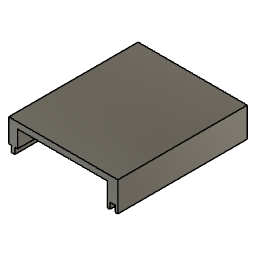
Headstage_dust_cover (Autodesk Fusion 360 design; units mm, degrees)
Autodesk Fusion 360 part; units mm, degrees
sketch "Sketch1" plane through (0, 22, 0) normal (0, 1, 0) x (-1, 0, 0)
  line L0 (11.5698, 0.25) -> (15.3, 0.25)
  line L1 (15.3, 0.25) -> (15.3, -0.5)
  line L2 (15.3, -0.5) -> (15.6004, -0.5)
  line L3 (15.6004, -0.5) -> (15.6004, -1.2)
  line L4 (15.6004, -1.2) -> (16.0004, -1.2)
  line L5 (16.0004, -1.2) -> (16.0004, -0.5)
  line L6 (16.0004, -0.5) -> (16.3, -0.5)
  line L7 (16.3, -0.5) -> (16.3, 1.05)
  line L8 (16.3, 1.05) -> (5, 1.05)
  line L9 (11.5698, -1.2) -> (11.5698, 0.25)
  line L10 (11.5698, -0.6208) -> (11.2698, -0.6208) construction
  line L11 (11.2698, -0.5) -> (11.2698, -1.2)
  line L12 (11.2698, -0.5) -> (10.5698, -0.5)
  line L13 (10.5698, -0.5) -> (10.5698, -1.2)
  line L14 (10.5698, -0.678) -> (10.2698, -0.678) construction
  line L15 (10.2698, 1.05) -> (10.2698, -1.2)
  line L16 (10.2698, 1.05) -> (16.3, 1.05)
  line L17 (16.3, -0.5) -> (16.0004, -0.5)
  line L18 (16.0004, -1.2) -> (15.6004, -1.2)
  line L19 (15.6004, -0.5) -> (15.3, -0.5)
  line L20 (15.3, 0.25) -> (11.5698, 0.25)
  line L21 (11.5698, -1.2) -> (11.2698, -1.2)
  line L22 (11.5698, -1.2) -> (11.2698, -1.2)
  line L23 (11.2698, -0.5) -> (10.5698, -0.5)
  line L24 (10.5698, -1.2) -> (10.2698, -1.2)
  line L25 (10.2698, 1.05) -> (16.3, 1.05)
  line L26 (16.3, -0.5) -> (16.0004, -0.5)
  line L27 (16.0004, -1.2) -> (15.6004, -1.2)
  line L28 (15.6004, -0.5) -> (15.3, -0.5)
  line L29 (15.3, 0.25) -> (11.5698, 0.25)
  dimension "d14" = 0.3
  dimension "d15" = 0.7
  dimension "d16" = 0.3
  constraint coincident L9 L10.start
  constraint perpendicular L9 L10
  constraint perpendicular L11 L12
  constraint coincident L13 L14.start
  constraint perpendicular L13 L14
  constraint coincident L8 L15.start
  constraint coincident L7.end L8.start
  constraint coincident L6.end L7.start
  constraint coincident L5.end L6.start
  constraint coincident L4.end L5.start
  constraint coincident L3.end L4.start
  constraint coincident L2.end L3.start
  constraint coincident L1.end L2.start
  constraint coincident L0.end L1.start
  constraint coincident L0.start L9.end
  constraint coincident L9.start L21.start
  constraint perpendicular L11 L21
  constraint perpendicular L13 L23
  constraint perpendicular L15 L24
  constraint perpendicular L7 L25
  measures "d14" distance of L10.start L10.end
  measures "d15" distance of L11.start L12.end
  measures "d16" distance of L14.start L14.end
extrude "Extrude1" add sketch "Sketch1" along normal blind 8.2 makes body 1
copy_body "Body->Comp1" bodies 1 removing the originals makes body 2 in component "Component"
move_face "OffsetFaces1" offset 0.3 1 faces at (-12.8132, 24.7333, 0.25) on bodies 2 in component "Component"
move_face "OffsetFaces2" offset -0.4 1 faces at (-12.2798, 27.4667, 1.05) on bodies 2 in component "Component"
move_face "OffsetFaces3" offset 3.3 1 faces at (-10.2698, 24.7333, 0.0333) on bodies 2 in component "Component"
move_face "OffsetFaces4" offset -3.3 1 faces at (-10.5698, 24.7333, -0.7333) on bodies 2 in component "Component"
move_face "OffsetFaces5" offset 3.3 1 faces at (-11.2698, 24.7333, -0.7333) on bodies 2 in component "Component"
move_face "OffsetFaces6" offset -3.3 1 faces at (-11.5698, 27.4667, -0.8167) on bodies 2 in component "Component"
move_face "OffsetFaces7" offset -4.2 1 faces at (-10.5132, 22, 0.4167) on bodies 2 in component "Component"
move_face "OffsetFaces8" offset -0.1 1 faces at (-8.2698, 28.8667, -0.4333) on bodies 2 in component "Component"
move_face "OffsetFaces9" offset 0.1 1 faces at (-7.9698, 27.5333, -0.7333) on bodies 2 in component "Component"
move_face "OffsetFaces10" offset 4.255 1 faces at (-10.4798, 26.2, 0.4167) on bodies 2 in component "Component"
move_face "OffsetFaces11" offset 0.3 1 faces at (-6.9698, 24.6967, 0.0333) on bodies 2 in component "Component"
move_face "OffsetFaces12" offset 0.3 1 faces at (-7.8698, 24.6967, -0.7333) on bodies 2 in component "Component"
move_face "OffsetFaces13" offset -0.3 1 faces at (-7.2698, 24.6967, -0.7333) on bodies 2 in component "Component"
move_face "OffsetFaces14" offset -0.3 1 faces at (-8.1698, 24.6967, -0.8167) on bodies 2 in component "Component"
move_face "OffsetFaces15" offset 2.77 1 faces at (-6.6698, 24.6967, 0.0333) on bodies 2 in component "Component"
move_face "OffsetFaces16" offset -2.77 1 faces at (-6.9698, 24.6967, -0.7333) on bodies 2 in component "Component"
move_face "OffsetFaces17" offset 2.77 1 faces at (-7.5698, 24.6967, -0.7333) on bodies 2 in component "Component"
move_face "OffsetFaces18" offset -2.77 1 faces at (-7.8698, 24.6967, -0.8167) on bodies 2 in component "Component"
move_face "OffsetFaces19" offset 6.445 1 faces at (-8.4332, 21.945, 0.4167) on bodies 2 in component "Component"
move_face "OffsetFaces20" offset 1.5 1 faces at (-12.1666, 20.4, 0.65) on bodies 2 in component "Component"
move_face "OffsetFaces21" offset -1.5 1 faces at (-8.4998, 20.4, -0.05) on bodies 2 in component "Component"
sketch "Sketch2" plane through (0, 0, 1.45) normal (0, 0, -1) x (1, 0, 0)
  line L0 (-5.0998, -15.5) -> (-15.3, -15.5)
  line L1 (-15.3, -15.5) -> (-15.3, -30.2)
  line L2 (-15.3, -30.2) -> (-5.0998, -30.2)
  line L3 (-5.0998, -30.2) -> (-5.0998, -15.5)
  line L4 (-5.0998, -15.5) -> (-5.0998, -26.3) construction
  line L5 (-5.0998, -26.3) -> (-15.3, -26.3)
  line L6 (-15.3, -26.3) -> (-15.3, -25.3)
  line L7 (-15.3, -25.3) -> (-5.0998, -25.3)
  line L8 (-5.0998, -25.3) -> (-5.0998, -26.3)
  dimension "d40" = 10.8
  dimension "d41" = 1
  constraint coincident L0.start L3.end
  constraint perpendicular L0 L4
  constraint horizontal L5
  constraint vertical L6
  constraint horizontal L7
  constraint vertical L8
  measures "d40" distance of L0.start L4.end
  measures "d41" distance of L4.end L7.end
extrude "Extrude1'" add sketch "Sketch2" along normal blind 1.5 contours L1 L3 L5 L6 L7 L8 bodies 2 in component "Component"
move_face "OffsetFaces22" offset 6 1 faces at (-11.8999, 25.3, 0.95) on bodies 2 in component "Component"
move_face "OffsetFaces23" offset -6 1 faces at (-8.4998, 26.3, 0.45) on bodies 2 in component "Component"
move_face "OffsetFaces24" offset 0.3 1 faces at (-8.4998, 20.3, 0.45) on bodies 2 in component "Component"
move_face "OffsetFaces25" offset -0.3 1 faces at (-8.4998, 19.3, 0.45) on bodies 2 in component "Component"
move_face "OffsetFaces26" offset -0.6 1 faces at (-8.4998, 19.6, 0.45) on bodies 2 in component "Component"
sketch "Sketch3" plane through (0, 0, 1.45) normal (0, 0, -1) x (1, 0, 0)
  line L0 (-5.0998, -20.6) -> (-15.3, -20.6)
  line L1 (-15.3, -20.6) -> (-15.3, -30.2)
  line L2 (-15.3, -30.2) -> (-5.0998, -30.2)
  line L3 (-5.0998, -30.2) -> (-5.0998, -20.6)
  line L4 (-5.0998, -30.2) -> (-8.3998, -30.2)
  line L5 (-8.3998, -30.2) -> (-8.3998, -29.8)
  line L6 (-8.3998, -29.8) -> (-5.0998, -29.8)
  line L7 (-5.0998, -29.8) -> (-5.0998, -30.2)
  line L8 (-15.3, -30.2) -> (-10.9, -30.2)
  line L9 (-10.9, -30.2) -> (-10.9, -29.8)
  line L10 (-10.9, -29.8) -> (-15.3, -29.8)
  line L11 (-15.3, -29.8) -> (-15.3, -30.2)
  dimension "d49" = 3.3
  dimension "d50" = 0.4
  dimension "d51" = 4.4
  dimension "d52" = 0.4
  constraint horizontal L4
  constraint vertical L5
  constraint horizontal L6
  constraint vertical L7
  constraint coincident L2.end L3.start
  constraint horizontal L8
  constraint vertical L9
  constraint horizontal L10
  constraint vertical L11
  constraint coincident L1.end L2.start
  measures "d49" distance of L2.end L4.end
  measures "d50" distance of L2.end L6.end
  measures "d51" distance of L1.end L8.end
  measures "d52" distance of L1.end L10.end
extrude "Extrude2" add sketch "Sketch3" along normal blind 1.95 contours L2 L3 L4 L5 L6 L7 | L1 L2 L8 L9 L10 L11 bodies 2 in component "Component"
move_face "OffsetFaces27" offset 0.45 1 faces at (-11.8999, 20.3333, -0.05) on bodies 2 in component "Component"
move_face "OffsetFaces28" offset -1.4 1 faces at (-10.9, 30.0667, 0.8) on bodies 2 in component "Component"
move_face "OffsetFaces29" offset 1.4 1 faces at (-8.3998, 30.0667, 0.8) on bodies 2 in component "Component"
component "Component" placed x (1, 0, 0) y (0, 1, 0) z (0, 0, 1) at (0, 0, 0)
